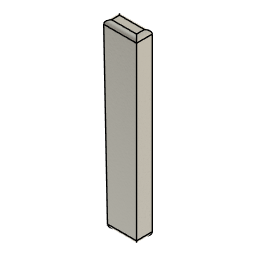
model (Autodesk Fusion 360 archive; units mm, degrees)
design "4"
part number: 2025-08-22-16-17-50-678
Autodesk Fusion 360 part; units mm, degrees
sketch "Sketch1" plane through (0, 0, 0) normal (0, 1, 0) x (1, 0, 0)
  line L0 (-20.0653, -74.6388) -> (4.9347, -74.6388)
  line L1 (4.9347, -74.6388) -> (4.9347, 61.3612)
  line L2 (4.9347, 61.3612) -> (-17.0653, 61.3612)
  line L3 (-17.0653, 61.3612) -> (-20.0653, -74.6388)
  dimension "d1" = 25
  dimension "d2" = 136
  dimension "d3" = 22
  constraint horizontal L0
  constraint perpendicular L0 L1
  constraint perpendicular L1 L2
  measures "d1" distance of L0.start L0.end
  measures "d2" distance of L0 L2
  measures "d3" distance of L1.end L2.end
extrude "Extrude1" add sketch "Sketch1" along normal blind 12
fillet "Fillet1" radius 3 1 faces at (-11.732, 4, 74.6388)
fillet "Fillet2" radius 3 1 faces at (-2.3987, 8, -61.3612)

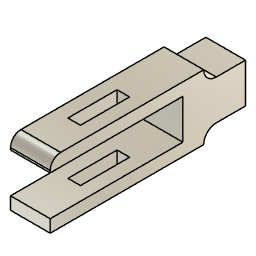
design "1"
part number: 2025-08-22-15-28-02-924
Autodesk Fusion 360 part; units mm, degrees
sketch "Sketch1" plane through (0, 0, 0) normal (1, 0, 0) x (0, 1, 0)
  line L0 (-85, 40) -> (-85, 28)
  line L1 (-85, 28) -> (42, 28)
  line L2 (-85, -10) -> (42, -10)
  line L3 (42, -10) -> (42, 28)
  line L4 (-85, 40) -> (62, 40)
  line L5 (62, 40) -> (62, -22)
  line L6 (62, -22) -> (-85, -22)
  line L7 (-85, -22) -> (-85, -10)
  dimension "d1" = 147
  dimension "d2" = 12
  dimension "d3" = 12
  dimension "d4" = 38
  dimension "d5" = 20
  dimension "d6" = 147
  constraint vertical L0
  constraint perpendicular L0 L1
  constraint perpendicular L0 L2
  constraint perpendicular L1 L3
  constraint perpendicular L0 L4
  constraint perpendicular L4 L5
  constraint perpendicular L5 L6
  constraint perpendicular L2 L7
  measures "d1" distance of L0.start L4.end
  measures "d2" distance of L0.start L0.end
  measures "d3" distance of L2.start L6.end
  measures "d4" distance of L1 L2
  measures "d5" distance of L3 L5
  measures "d6" distance of L5.end L6.end
extrude "Extrude1" add sketch "Sketch1" along normal blind 38
sketch "Sketch2" plane through (0, 0, 40) normal (0, 0, 1) x (-1, 0, 0)
  line L0 (0, -62) -> (0, 85)
  line L1 (0, 85) -> (-38, 85)
  line L2 (-38, 85) -> (-38, -62)
  line L3 (-38, -62) -> (0, -62)
  line L4 (-13, -4) -> (-25, -4)
  line L5 (-25, -4) -> (-25, 43)
  line L6 (-25, 43) -> (-13, 43)
  line L7 (-13, 43) -> (-13, -4)
  line L8 (-13, -4) -> (-25, 43) construction
  line L9 (-25, -4) -> (-13, 43) construction
  point P0 (-19, 19.5)
  dimension "d9" = 12
  dimension "d10" = 47
  dimension "d11" = 19
  dimension "d12" = 58
  constraint horizontal L4
  constraint perpendicular L4 L5
  constraint parallel L4 L6
  constraint parallel L5 L7
  constraint coincident L8 P0
  constraint coincident L9 P0
  measures "d9" distance of L5.end L6.end
  measures "d10" distance of L4.start L6.end
  measures "d11" distance of L2 P0
  measures "d12" distance of L3 L4
extrude "Extrude2" cut sketch "Sketch2" along normal through all and the other way through all contours L4 L5 L6 L7
sketch "Sketch3" plane through (0, 62, 0) normal (0, 1, 0) x (-1, 0, 0)
  line L0 (0, -22) -> (0, 40)
  line L1 (0, 40) -> (-38, 40)
  line L2 (-38, 40) -> (-38, -22)
  line L3 (-38, -22) -> (0, -22)
  line L4 (0, 28) -> (-38, 28)
  line L5 (-38, 28) -> (-38, -10)
  line L6 (-38, -10) -> (0, -10)
  line L7 (0, -10) -> (0, 28)
  line L8 (0, 28) -> (-38, -10) construction
  line L9 (-38, 28) -> (0, -10) construction
  point P0 (-19, 9)
  dimension "d14" = 38
  dimension "d15" = 38
  dimension "d16" = 31
  constraint horizontal L4
  constraint perpendicular L4 L5
  constraint parallel L4 L6
  constraint parallel L5 L7
  constraint coincident L8 P0
  constraint coincident L9 P0
  measures "d14" distance of L4.start L4.end
  measures "d15" distance of L4.end L5.end
  measures "d16" distance of L3 P0
extrude "Extrude3" add sketch "Sketch3" along normal blind 40 contours L0 L2 L4 L5 L6 L7
fillet "Fillet1" radius 12 1 edges at (19, 62, 28)
fillet "Fillet2" radius 12 1 edges at (19, 62, -10)
fillet "Fillet3" radius 10 1 edges at (19, -85, 40)

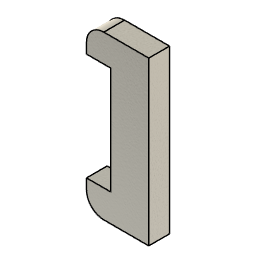
design "3"
part number: 2025-08-22-16-09-13-701
Autodesk Fusion 360 part; units mm, degrees
sketch "Sketch1" plane through (0, 0, 0) normal (0, 1, 0) x (1, 0, 0)
  line L0 (-50, -55) -> (-50, -39)
  line L1 (-50, -39) -> (-36, -39)
  line L2 (-36, -39) -> (-36, 23)
  line L3 (-36, 23) -> (-50, 23)
  line L4 (-50, 23) -> (-50, 39)
  line L5 (-50, 39) -> (-14, 39)
  line L6 (-50, -55) -> (-14, -55)
  line L7 (-14, -55) -> (-14, 39)
  dimension "d1" = 16
  dimension "d2" = 16
  dimension "d3" = 22
  dimension "d4" = 62
  dimension "d5" = 14
  constraint vertical L0
  constraint perpendicular L0 L1
  constraint perpendicular L1 L2
  constraint perpendicular L0 L3
  constraint perpendicular L1 L4
  constraint perpendicular L4 L5
  constraint perpendicular L0 L6
  constraint perpendicular L5 L7
  constraint collinear L0 L4
  measures "d1" distance of L0.start L0.end
  measures "d2" distance of L3.end L4.end
  measures "d3" distance of L2 L7
  measures "d4" distance of L1 L3
  measures "d5" distance of L2.end L3.end
extrude "Extrude1" add sketch "Sketch1" along normal blind 12
fillet "Fillet1" radius 10 1 edges at (-50, 6, 55)
fillet "Fillet2" radius 10 1 edges at (-50, 6, -39)

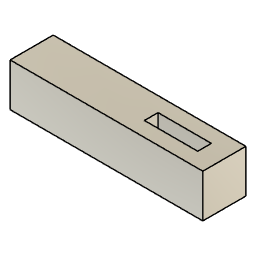
design "2"
part number: 2025-08-22-16-01-23-106
Autodesk Fusion 360 part; units mm, degrees
sketch "Sketch1" plane through (0, 0, 0) normal (1, 0, 0) x (0, 1, 0)
  line L0 (-30.526, 19.0055) -> (-68.526, 19.0055)
  line L1 (-68.526, 19.0055) -> (-68.526, 57.0055)
  line L2 (-68.526, 57.0055) -> (-30.526, 57.0055)
  line L3 (-30.526, 57.0055) -> (-30.526, 19.0055)
  line L4 (-30.526, 19.0055) -> (-68.526, 57.0055) construction
  line L5 (-68.526, 19.0055) -> (-30.526, 57.0055) construction
  point P0 (-49.526, 38.0055)
  dimension "d1" = 38
  dimension "d2" = 38
  constraint horizontal L0
  constraint perpendicular L0 L1
  constraint parallel L0 L2
  constraint parallel L1 L3
  constraint coincident L4 P0
  constraint coincident L5 P0
  measures "d1" distance of L1.end L2.end
  measures "d2" distance of L0.start L2.end
extrude "Extrude1" add sketch "Sketch1" along normal blind 170
sketch "Sketch2" plane through (0, 0, 57.0055) normal (0, 0, 1) x (-1, 0, 0)
  line L0 (0, 30.526) -> (0, 68.526)
  line L1 (0, 68.526) -> (-170, 68.526)
  line L2 (-170, 68.526) -> (-170, 30.526)
  line L3 (-170, 30.526) -> (0, 30.526)
  line L4 (-152.5, 55.526) -> (-105.5, 55.526)
  line L5 (-105.5, 55.526) -> (-105.5, 43.526)
  line L6 (-105.5, 43.526) -> (-152.5, 43.526)
  line L7 (-152.5, 43.526) -> (-152.5, 55.526)
  line L8 (-152.5, 55.526) -> (-105.5, 43.526) construction
  line L9 (-105.5, 55.526) -> (-152.5, 43.526) construction
  point P0 (-129, 49.526)
  dimension "d5" = 12
  dimension "d6" = 47
  dimension "d7" = 41
  dimension "d8" = 19
  constraint horizontal L4
  constraint perpendicular L4 L5
  constraint parallel L4 L6
  constraint parallel L5 L7
  constraint coincident L8 P0
  constraint coincident L9 P0
  measures "d5" distance of L4.start L6.end
  measures "d6" distance of L4.start L4.end
  measures "d7" distance of L2 P0
  measures "d8" distance of L1 P0
extrude "Extrude2" cut sketch "Sketch2" along normal through all and the other way through all contours L4 L5 L6 L7
